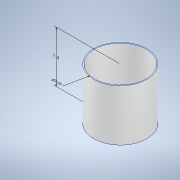
# Autodesk Inventor part: HP-01
Saved by Autodesk Inventor 2022 (Build 260153000, 153)
## iProperties
Company: El Camino College
Created: 2023-05-12
Part Number: HP-01
Material: Aluminum 6061
Document SubType Name: Modeling
Designer: Edgar Tejada
Density: 2.7 g/cm^3
Appearance: Aluminum - Flat
Mass: 1158.24 g
Surface Area: 2707.35 cm^2
Volume: 428.979 cm^3
Project: Hexagonal Hive
Description: Hotpot for Melting Wax
Author: Edgar Tejada
Title: Hot Pot
Autodesk Inventor part; units mm, degrees
ref_plane "YZ Plane" through (0, 0, 0) normal (1, 0, 0) x (0, 1, 0)
ref_plane "XZ Plane" through (0, 0, 0) normal (0, 1, 0) x (-1, 0, 0)
ref_plane "XY Plane" through (0, 0, 0) normal (0, 0, 1) x (1, 0, 0)
sketch "Sketch1" plane through (0, 0, 0) normal (0, 1, 0) x (-1, 0, 0)
  circle A0 centre (0, 0) radius 95.25
  dimension "d0" = 190.5
  constraints: 1 centre point, 1 coincident
  measures "d0" diameter of A0
extrude "Extrusion1" add sketch "Sketch1" along normal blind 184.15
shell "Shell1" thickness 3.175 removed faces 0
sketch "Sketch2" plane through (0, 184.15, 0) normal (0, 1, 0) x (1, 0, 0)
  circle A0 centre (0, 0) radius 92.075
  circle A1 centre (0, 0) radius 95.25 projected
  dimension "d4" = 3.175
  constraints: 1 centre point, 1 coincident
  measures "d4" radial gap between concentric circles of A1 A0
extrude "Extrusion2" cut sketch "Sketch2" against normal up to next contours A0
fillet "Fillet1" radius 3.175 1 edges at (92.075, 3.175, 0)
sketch "Sketch3" plane through (0, -30.1625, 0) normal (0, 0, 1) x (1, 0, 0)
  circle A0 centre (0, 55.5625) radius 9.525
  line L0 (120.65, 30.1625) -> (-120.65, 30.1625)
  point P0 (0, 30.1625)
  point P1 (0, 30.1625)
  point P2 (0, 30.1625)
  dimension "d12" = 19.05
  dimension "d11" = 25.4
  dimension "d16" = 0
  constraints: 2 end point, 1 centre point, 1 coincident, 1 midpoint, 1 vertical alignment
  measures "d12" diameter of A0
  measures "d11" distance of point (0, 30.163) A0.centre
  measures "d16" distance of point (0, 30.163) point (0, 30.163)
extrude "Extrusion3" cut sketch "Sketch3" against normal through all
equation "\"d4\" = d3"
equation "\"d7\" = d3"
equation "\"d3\" = 3.175"
body "Solid1"
